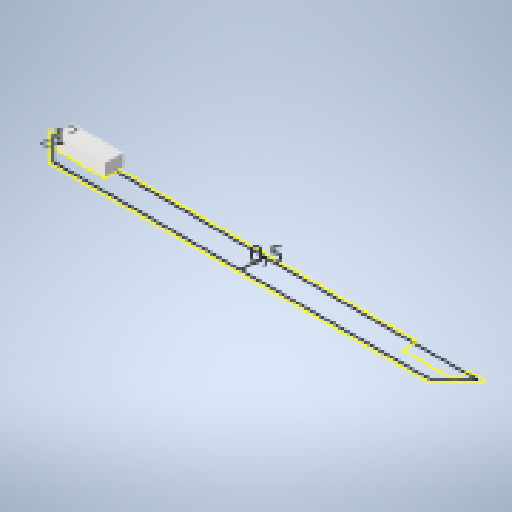
# Autodesk Inventor part: microswitch_cap
Saved by Autodesk Inventor 2025 (Build 290162000, 162)
## iProperties
Created: 2026-08-07
Part Number: microswitch_cap
Material: Типовые
Document SubType Name: Modeling
Designer: garin
Density: 1 g/cm^3
Appearance: По умолчанию
Author: garin
Autodesk Inventor part; units mm, degrees
ref_plane "YZ Plane" through (0, 0, 0) normal (1, 0, 0) x (0, 1, 0)
ref_plane "XZ Plane" through (0, 0, 0) normal (0, 1, 0) x (-1, 0, 0)
ref_plane "XY Plane" through (0, 0, 0) normal (0, 0, 1) x (1, 0, 0)
sketch "Эскиз1" plane through (0, 0, 0) normal (0, 1, 0) x (-1, 0, 0)
  line L0 (-7.5, 2.8) -> (7.5, 2.8)
  line L1 (7.5, 2.8) -> (7.5, -2.8)
  line L2 (7.5, -2.8) -> (-7.5, -2.8)
  line L3 (-7.5, -2.8) -> (-7.5, 2.8)
  line L4 (-7.5, 2.8) -> (7.5, -2.8) construction
  line L5 (7.5, 2.8) -> (-7.5, -2.8) construction
  point P0 (0, 0)
  dimension "d0" = 15
  dimension "d1" = 5.6
  constraints: 12 end point, 2 midpoint, 2 parallel, 1 horizontal, 1 perpendicular
  measures "d0" distance of L1.end L2.end
  measures "d1" distance of L0.end L1.end
extrude "Выдавливание1" add sketch "Эскиз1" along normal blind 5.6
chamfer "Фаска1" distance 1 angle 45 1 edges at (-7.5, 2.8, 2.8)
sketch "Эскиз2" plane through (0, 0, 0) normal (0, -1, 0) x (1, 0, 0)
  line L0 (112.65, -2) -> (112.65, 2) projected
  line L1 (112.65, -2) -> (118.15, -2) projected
  line L2 (118.15, -2) -> (118.15, -0.4142) projected
  line L3 (118.15, -0.4142) -> (109.7358, 8) projected
  line L4 (109.7358, 8) -> (-4.8358, 8) projected
  line L5 (-4.8358, 8) -> (-13.25, -0.4142) projected
  line L6 (-13.25, -0.4142) -> (-13.25, -2) projected
  line L7 (-13.25, -2) -> (-7.75, -2) projected
  line L8 (-7.75, 2) -> (-7.75, -2) projected
  line L9 (-6.75, 3) -> (-7.75, 2) projected
  line L10 (7.75, 3) -> (-6.75, 3) projected
  line L11 (7.75, -2) -> (7.75, 3) projected
  line L12 (7.75, -2) -> (97.15, -2) projected
  line L13 (97.15, 3) -> (97.15, -2) projected
  line L14 (111.65, 3) -> (97.15, 3) projected
  line L15 (112.65, 2) -> (111.65, 3) projected
  line L16 (52.45, 8) -> (52.45, -2) construction
  line L17 (-9.25, -1) -> (-12.4216, -1)
  line L18 (-12.4216, -1) -> (-4.4216, 7)
  line L19 (-4.4216, 7) -> (109.3216, 7)
  line L20 (109.3216, 7) -> (117.3216, -1)
  line L21 (-9.25, -1) -> (117.3216, -1)
  line L22 (52.45, 7) -> (51.95, 7) construction
  line L23 (51.95, 7) -> (51.95, -1)
  line L24 (51.95, -1) -> (52.45, -1) construction
  line L25 (52.45, -1) -> (52.45, 7) construction
  point P0 (0, 0)
  point P1 (51.95, 7)
  dimension "d7" = 1
  dimension "d8" = 0.5
  constraints: 20 end point, 3 midpoint, 3 parallel, 1 horizontal, 1 perpendicular, 1 point on line, 3 other
  measures "d7" distance between parallel lines of L7 L17
  measures "d8" distance of L24.end L23.end
extrude "Выдавливание2" add sketch "Эскиз2" against normal blind 1.6 contours L21 L11 L10 L9 L8 L17 L18 L19 L23 | L21 L8 L9 L10 L11
